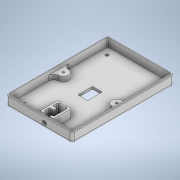
# Autodesk Inventor part: Controller_Back
Saved by Autodesk Inventor 2022.3 (Build 263350000, 350)
## iProperties
Created: 2023-06-20
Part Number: Controller_Back
Material: Generic
Document SubType Name: Modeling
Designer: natalie.jimenez
Density: 1 g/cm^3
Appearance: Default
Author: natalie.jimenez
Autodesk Inventor part; units mm, degrees
note: some values were not read from the file. Chosen so that the rebuilt part matches the saved one: direction of "Hole5"; direction of "Hole6".
ref_plane "YZ Plane" through (0, 0, 0) normal (1, 0, 0) x (0, 1, 0)
ref_plane "XZ Plane" through (0, 0, 0) normal (0, 1, 0) x (-1, 0, 0)
ref_plane "XY Plane" through (0, 0, 0) normal (0, 0, 1) x (1, 0, 0)
sketch "Sketch1" plane through (0, 0, 0) normal (0, 1, 0) x (-1, 0, 0)
  line L0 (40.64, -63.5) -> (-40.64, -63.5)
  line L1 (-40.64, -63.5) -> (-40.64, 63.5)
  line L2 (-40.64, 63.5) -> (40.64, 63.5)
  line L3 (40.64, 63.5) -> (40.64, -63.5)
  line L4 (40.64, -63.5) -> (-40.64, 63.5) construction
  line L5 (-40.64, -63.5) -> (40.64, 63.5) construction
  point P0 (0, 0)
  dimension "d0" = 127
  dimension "d1" = 81.28
  constraints: 12 end point, 2 midpoint, 2 parallel, 1 horizontal, 1 perpendicular
  measures "d0" distance between parallel lines of L0 L2
  measures "d1" distance between parallel lines of L1 L3
extrude "Extrusion1" add sketch "Sketch1" along normal blind 3.175
sketch "Sketch16" plane through (0, 0, 0) normal (0, -1, 0) x (1, 0, 0)
  line L0 (-42.672, -65.532) -> (42.672, -65.532)
  line L1 (42.672, -65.532) -> (42.672, 65.532)
  line L2 (42.672, 65.532) -> (-42.672, 65.532)
  line L3 (-42.672, 65.532) -> (-42.672, -65.532)
  line L4 (40.64, -63.5) -> (-40.64, -63.5) projected
  line L5 (-40.64, 63.5) -> (40.64, 63.5) projected
  line L6 (-40.64, -63.5) -> (-40.64, 63.5) projected
  line L7 (40.64, 63.5) -> (40.64, -63.5) projected
  point P0 (0, 0)
  dimension "d99" = 2.032
  dimension "d100" = 2.032
  dimension "d101" = 2.032
  dimension "d102" = 2.032
  constraints: 8 end point, 2 parallel, 1 horizontal, 1 perpendicular
  measures "d99" distance between parallel lines of L4 L0
  measures "d100" distance between parallel lines of L2 L5
  measures "d101" distance between parallel lines of L3 L6
  measures "d102" distance between parallel lines of L1 L7
extrude "Extrusion9" add sketch "Sketch16" against normal blind 12.7
fillet "Fillet1" radius 3.175 8 edges at (-42.672, 0, 0) (0, 0, 65.532) (42.672, 0, 0) (0, 0, -65.532) (-42.672, 6.35, -65.532) (42.672, 6.35, -65.532) (-42.672, 6.35, 65.532) (42.672, 6.35, 65.532)
fillet "Fillet3" radius 1.143 4 edges at (-40.64, 7.9375, -63.5) (40.64, 7.9375, -63.5) (-40.64, 7.9375, 63.5) (40.64, 7.9375, 63.5)
sketch "Sketch19" plane through (0, 12.7, 0) normal (0, 1, 0) x (1, 0, 0)
  arc A0 (-40.64, -62.357) -> (-39.497, -63.5) centre (-39.497, -62.357) ccw projected
  line L0 (39.497, -63.5) -> (-39.497, -63.5) projected
  line L1 (-40.64, -62.357) -> (-40.64, 62.357) projected
  arc A1 (-39.497, 63.5) -> (-40.64, 62.357) centre (-39.497, 62.357) ccw projected
  line L2 (-39.497, 63.5) -> (39.497, 63.5) projected
  arc A2 (40.64, 62.357) -> (39.497, 63.5) centre (39.497, 62.357) ccw projected
  line L3 (40.64, 62.357) -> (40.64, -62.357) projected
  arc A3 (39.497, -63.5) -> (40.64, -62.357) centre (39.497, -62.357) ccw projected
  line L4 (-41.656, 62.357) -> (-41.656, -62.357)
  arc A4 (-41.656, -62.357) -> (-39.497, -64.516) centre (-39.497, -62.357) ccw
  line L5 (-39.497, -64.516) -> (39.497, -64.516)
  arc A5 (39.497, -64.516) -> (41.656, -62.357) centre (39.497, -62.357) ccw
  line L6 (41.656, -62.357) -> (41.656, 62.357)
  arc A6 (41.656, 62.357) -> (39.497, 64.516) centre (39.497, 62.357) ccw
  line L7 (39.497, 64.516) -> (-39.497, 64.516)
  arc A7 (-39.497, 64.516) -> (-41.656, 62.357) centre (-39.497, 62.357) ccw
  point P0 (0, 0)
  dimension "d127" = 1.016
  constraints: 8 end point, 8 point on circle, 4 centre point, 7 other
  measures "d127" distance between parallel lines of L1 L4
extrude "Extrusion12" add sketch "Sketch19" along normal blind 1.27
sketch "Sketch20" plane through (0, 0, 0) normal (0, -1, 0) x (1, 0, 0)
  line L0 (-31.75, -53.721) -> (31.75, -53.721) construction
  line L1 (31.75, -53.721) -> (31.75, 53.721) construction
  line L2 (31.75, 53.721) -> (-31.75, 53.721) construction
  line L3 (-31.75, 53.721) -> (-31.75, -53.721) construction
  line L4 (-31.75, -53.721) -> (31.75, 53.721) construction
  line L5 (31.75, -53.721) -> (-31.75, 53.721) construction
  point P0 (0, 0)
  point P1 (31.75, -25.781)
  point P2 (31.75, 31.369)
  dimension "d130" = 57.15
  dimension "d131" = 63.5
  dimension "d132" = 107.442
  dimension "d207" = 27.94
  constraints: 12 end point, 2 coincident, 2 midpoint, 2 parallel, 2 point on line, 1 horizontal, 1 perpendicular
  measures "d130" distance of point (31.75, -25.781) point (31.75, 31.369)
  measures "d131" distance between parallel lines of L1 L3
  measures "d132" distance of point (-31.75, -53.721) L2.end
  measures "d207" vertical distance of point (31.75, -25.781) point (-31.75, -53.721)
sketch "Sketch21" plane through (0, 0, 0) normal (0, -1, 0) x (1, 0, 0)
  line L0 (-6.35, -9.525) -> (6.35, -9.525)
  line L1 (6.35, -9.525) -> (6.35, 9.525)
  line L2 (6.35, 9.525) -> (-6.35, 9.525)
  line L3 (-6.35, 9.525) -> (-6.35, -9.525)
  line L4 (-6.35, -9.525) -> (6.35, 9.525) construction
  line L5 (6.35, -9.525) -> (-6.35, 9.525) construction
  point P0 (0, 0)
  dimension "d133" = 12.7
  dimension "d134" = 19.05
  constraints: 12 end point, 2 midpoint, 2 parallel, 1 horizontal, 1 perpendicular
  measures "d133" distance between parallel lines of L1 L3
  measures "d134" distance between parallel lines of L0 L2
hole "Hole5" at (-31.75, 0, -53.721) at (31.75, 0, -25.781) at (31.75, 0, 31.369) at (-31.75, 0, 53.721) direction (0, 1, 0) diameter 3.81 depth 3.175 clearance for "Flat Head Machine Screw (82)" size "#6" standard "Ansi Unified Screw Threads"
extrude "Extrusion13" cut sketch "Sketch21" against normal up to surface (3.175 mm away)
fillet "Fillet4" radius 1.143 4 edges at (6.35, 1.5875, -9.525) (6.35, 1.5875, 9.525) (-6.35, 1.5875, 9.525) (-6.35, 1.5875, -9.525)
sketch "Sketch22" plane through (0, 0, 0) normal (0, -1, 0) x (1, 0, 0)
  line L0 (40.64, 62.357) -> (40.64, -62.357) projected
  line L1 (-40.64, -62.357) -> (-40.64, 62.357) projected
  line L2 (-59.7408, 0) -> (59.7408, 0) projected
  point P0 (0, 0)
  point P1 (34.29, 0)
  point P2 (-34.29, 0)
  point P3 (40.64, 0)
  point P4 (-40.64, 0)
  dimension "d147" = 6.35
  dimension "d148" = 6.35
  constraints: 2 midpoint, 2 point on line
  measures "d147" distance of point (40.64, 0) point (34.29, 0)
  measures "d148" distance of point (-34.29, 0) point (-40.64, 0)
hole "Hole6" at (-34.29, 0, 0) at (34.29, 0, 0) direction (0, 1, 0) diameter 2.6416 depth 3.175 thread size "6-32 UNC" class "2B" standard "ANSI Unified Screw Threads"
sketch "Sketch24" plane through (-39.497, 12.7, 65.532) normal (0, 0, 1) x (1, 0, 0)
  circle A0 centre (46.029, -6.6675) radius 2.8575
  line L0 (0, 0) -> (78.994, 0) projected
  line L1 (78.994, -9.525) -> (0, -9.525) projected
  line L2 (0, 0) -> (78.994, 0) projected
  line L3 (78.994, 0) -> (78.994, -9.525) projected
  point P0 (39.497, -12.7)
  point P1 (78.994, -4.7625)
  dimension "d157" = 5.715
  dimension "d159" = 33.02
  constraints: 1 centre point, 1 midpoint, 1 tangent
  measures "d157" diameter of A0
  measures "d159" distance of point (78.994, -4.763) A0.centre
extrude "Extrusion14" cut sketch "Sketch24" against normal up to surface (2.032 mm away)
sketch "Sketch25" plane through (0, 3.175, 0) normal (0, 1, 0) x (1, 0, 0)
  line L0 (3.6745, -63.5) -> (9.3895, -63.5) projected
  line L1 (-39.497, -62.357) -> (39.497, -62.357) projected
  line L2 (10.0245, -62.357) -> (15.7395, -62.357)
  line L3 (15.7395, -62.357) -> (15.7395, -39.497)
  line L4 (-2.0405, -39.497) -> (3.0395, -39.497)
  line L5 (15.7395, -62.357) -> (15.7395, -39.497)
  line L6 (-2.0405, -62.357) -> (-2.0405, -39.497)
  line L7 (15.7395, -39.497) -> (10.0245, -39.497)
  line L8 (10.0245, -39.497) -> (10.0245, -42.037)
  line L9 (10.0245, -42.037) -> (13.1995, -42.037)
  line L10 (0.4995, -42.037) -> (3.0395, -42.037)
  line L11 (3.0395, -42.037) -> (3.0395, -39.497)
  line L12 (15.7395, -62.357) -> (10.0245, -62.357)
  line L13 (10.0245, -62.357) -> (10.0245, -59.817)
  line L14 (10.0245, -59.817) -> (13.1995, -59.817)
  line L15 (3.0395, -62.357) -> (3.0395, -59.817)
  line L16 (3.0395, -59.817) -> (0.4995, -59.817)
  line L17 (0.4995, -52.832) -> (6.2145, -52.832)
  line L18 (6.2145, -52.832) -> (6.2145, -49.022)
  line L19 (6.2145, -49.022) -> (0.4995, -49.022)
  line L20 (39.497, -62.357) -> (39.497, 62.357) projected
  line L21 (15.7395, -39.497) -> (15.7395, -62.357)
  line L22 (10.0245, -62.357) -> (10.0245, -59.817)
  line L23 (0.4995, -49.022) -> (0.4995, -42.037)
  line L24 (0.4995, -52.832) -> (0.4995, -59.817)
  line L25 (10.0245, -40.767) -> (15.7395, -40.767) construction
  line L26 (10.0245, -61.087) -> (15.7395, -61.087) construction
  line L27 (13.1995, -42.037) -> (13.1995, -59.817)
  line L28 (-2.0405, -62.357) -> (3.0395, -62.357)
  line L29 (10.0245, -61.087) -> (3.0395, -61.087) construction
  line L30 (6.532, -63.5) -> (6.532, -61.087) construction
  point P0 (0, 0)
  point P1 (0.4995, -39.497)
  point P2 (12.882, -39.497)
  point P3 (-2.0405, -50.927)
  point P4 (0.4995, -56.3245)
  point P5 (3.0395, -40.767)
  dimension "d168" = 2.54
  dimension "d175" = 6.985
  dimension "d179" = 3.81
  dimension "d180" = 6.985
  dimension "d184" = 6.985
  dimension "d186" = 6.985
  dimension "d188" = 6.985
  dimension "d190" = 5.08
  dimension "d191" = 2.54
  dimension "d192" = 6.985
  dimension "d193" = 12.7
  dimension "d195" = 2.54
  dimension "d196" = 2.54
  dimension "d197" = 2.54
  constraints: 59 end point, 13 perpendicular, 10 midpoint, 8 parallel, 6 point on line, 4 horizontal, 2 collinear, 1 coincident, 2 other
  measures "d168" distance from line of L10 point (0.499, -39.497)
  measures "d175" distance between parallel lines of L8 L11
  measures "d179" distance between parallel lines of L17 L19
  measures "d180" distance of L26.start L29.end
  measures "d184" distance between parallel lines of L19 L10
  measures "d186" distance from line of L14 L17.end
  measures "d188" distance from line of L19 L8.end
  measures "d190" distance from line of point (3.039, -40.767) L6
  measures "d191" distance between parallel lines of L24 L6
  measures "d192" distance between parallel lines of L27 L18
  measures "d193" distance between parallel lines of L23 L27
  measures "d195" distance between parallel lines of L9 L7
  measures "d196" distance between parallel lines of L2 L14
  measures "d197" distance between parallel lines of L5 L27
extrude "Extrusion15" add sketch "Sketch25" along normal up to surface (10.795 mm away)
fillet "Fillet5" radius 1.27 20 edges at (15.7395, 8.5725, 39.497) (-2.0405, 8.5725, 39.497) (15.7395, 8.5725, 62.357) (-2.0405, 8.5725, 62.357) (6.2145, 8.5725, 49.022) (6.2145, 8.5725, 52.832) (0.4995, 8.5725, 42.037) (0.4995, 8.5725, 59.817) (13.1995, 8.5725, 59.817) (10.0245, 8.5725, 42.037) (10.0245, 8.5725, 39.497) (13.1995, 8.5725, 42.037) (10.0245, 8.5725, 59.817) (10.0245, 8.5725, 62.357) (3.0395, 8.5725, 42.037) (3.0395, 8.5725, 39.497) (3.0395, 8.5725, 59.817) (3.0395, 8.5725, 62.357) (0.4995, 8.5725, 52.832) (0.4995, 8.5725, 49.022)
sketch "Sketch26" plane through (0, 3.175, 0) normal (0, 1, 0) x (1, 0, 0)
  circle A0 centre (34.29, 0) radius 1.3208 projected
  arc A1 (34.29, 6.35) -> (34.29, -6.35) centre (34.29, 0) ccw
  circle A2 centre (-34.29, 0) radius 1.3208 projected
  arc A3 (-34.29, -6.35) -> (-34.29, 6.35) centre (-34.29, 0) ccw
  line L0 (40.64, -62.357) -> (40.64, 62.357) projected
  arc A4 (34.29, 6.35) -> (40.64, 12.7) centre (34.29, 12.7) ccw
  line L1 (-40.64, 62.357) -> (-40.64, -62.357) projected
  arc A5 (-40.64, 12.7) -> (-34.29, 6.35) centre (-34.29, 12.7) ccw
  line L2 (59.7408, 0) -> (-59.7408, 0) projected
  arc A6 (40.64, -12.7) -> (34.29, -6.35) centre (34.29, -12.7) ccw
  arc A7 (-34.29, -6.35) -> (-40.64, -12.7) centre (-34.29, -12.7) ccw
  point P0 (0, 0)
  point P1 (-40.64, -12.7)
  point P2 (40.64, -12.7)
  dimension "d201" = 12.7
  dimension "d202" = 12.7
  dimension "d203" = 6.35
  dimension "d204" = 6.35
  constraints: 12 point on circle, 6 centre point, 6 symmetric about line, 4 tangent, 2 coincident, 2 point on line, 2 other
  measures "d201" diameter of A3
  measures "d202" diameter of A1
  measures "d203" radius of A4
  measures "d204" radius of A5
extrude "Extrusion16" add sketch "Sketch26" along normal blind 6.35 contours L2 L0 A6 A1 A0 | A0 L2 A1 A4 L0 | L2 A3 A7 L1 A2 | A2 L2 L1 A5 A3
sketch "Sketch2" plane through (0, 3.175, 0) normal (0, 1, 0) x (1, 0, 0)
  line L0 (11.7475, 17.4625) -> (-11.7475, 17.4625)
  line L1 (-11.7475, 17.4625) -> (-11.7475, -17.4625)
  line L2 (-11.7475, -17.4625) -> (11.7475, -17.4625)
  line L3 (11.7475, -17.4625) -> (11.7475, 17.4625)
  line L4 (11.7475, 17.4625) -> (-11.7475, -17.4625) construction
  line L5 (-11.7475, 17.4625) -> (11.7475, -17.4625) construction
  point P0 (0, 0)
  dimension "d4" = 23.495
  dimension "d5" = 34.925
  constraints: 12 end point, 2 midpoint, 2 parallel, 1 horizontal, 1 perpendicular
  measures "d4" distance between parallel lines of L3 L1
  measures "d5" distance between parallel lines of L0 L2
sketch "Sketch4" plane through (0, 0, 0) normal (0, 0, 1) x (1, 0, 0)
  line L0 (11.7475, 1.143) -> (17.3304, 3.175)
  line L1 (40.64, 3.175) -> (-40.64, 3.175) projected
  line L2 (11.7475, 3.175) -> (11.7475, 1.143) projected
  line L3 (11.7475, 1.143) -> (11.7475, 3.175)
  line L4 (11.7475, 3.175) -> (17.3304, 3.175)
  point P0 (0, 0)
  dimension "d8" = 70
  constraints: 6 end point, 1 collinear, 1 perpendicular, 1 point on line
  measures "d8" angle of L2 L0
sketch "Sketch5" plane through (0, 0, 0) normal (0, 0, 1) x (1, 0, 0)
  line L0 (-11.7475, 1.143) -> (11.7475, 1.143) projected
  line L1 (40.64, 3.175) -> (-40.64, 3.175) projected
  line L2 (-11.7475, 1.143) -> (-16.8275, 1.143)
  line L3 (-16.8275, 1.143) -> (-16.8275, 3.175)
  line L4 (-16.8275, 3.175) -> (-11.7475, 3.175)
  line L5 (-11.7475, 3.175) -> (-11.7475, 1.143)
  point P0 (0, 0)
  point P1 (-11.7475, 2.159)
  point P2 (-16.8275, 2.159)
  dimension "d11" = 5.08
  constraints: 8 end point, 2 midpoint, 2 parallel, 1 horizontal, 1 perpendicular, 1 point on line
  measures "d11" distance of point (-11.748, 2.159) point (-16.828, 2.159)
sketch "Sketch6" plane through (0, 1.143, 0) normal (0, 1, 0) x (1, 0, 0)
  line L0 (-11.7475, -17.4625) -> (-11.7475, -7.62) projected
  line L1 (11.7475, -17.4625) -> (-11.7475, -17.4625) projected
  line L2 (11.7475, -7.62) -> (11.7475, -17.4625) projected
  line L3 (11.7475, 7.62) -> (11.7475, -7.62) projected
  line L4 (11.7475, 17.4625) -> (11.7475, 7.62) projected
  line L5 (-11.7475, 17.4625) -> (11.7475, 17.4625) projected
  line L6 (-11.7475, 7.62) -> (-11.7475, 17.4625) projected
  line L7 (-11.7475, 7.62) -> (-16.8275, 7.62) projected
  line L8 (-16.8275, 7.62) -> (-16.8275, -7.62) projected
  line L9 (-16.8275, -7.62) -> (-11.7475, -7.62) projected
  line L10 (-10.6045, 16.0655) -> (6.9215, 16.0655)
  line L11 (6.9215, 16.0655) -> (6.9215, -16.0655)
  line L12 (6.9215, -16.0655) -> (-10.6045, -16.0655)
  line L13 (-10.6045, -16.0655) -> (-10.6045, 16.0655)
  line L14 (11.7475, 7.62) -> (11.7475, -7.62) projected
  line L15 (11.7475, 0) -> (-16.8275, 0) construction
  line L16 (-16.8275, -7.62) -> (-16.8275, 7.62) projected
  line L17 (6.9215, 0) -> (-10.6045, 0) construction
  point P0 (0, 0)
  dimension "d14" = 17.526
  dimension "d15" = 32.131
  dimension "d16" = 4.826
  constraints: 12 end point, 4 midpoint, 2 parallel, 1 collinear, 1 horizontal, 1 perpendicular
  measures "d14" distance between parallel lines of L11 L13
  measures "d15" distance between parallel lines of L12 L10
  measures "d16" distance between parallel lines of L3 L11
sketch "Sketch7" plane through (0, 3.175, 0) normal (0, 1, 0) x (1, 0, 0)
  line L0 (-14.2875, 12.7) -> (13.6525, 12.7) construction
  line L1 (13.6525, 12.7) -> (13.6525, -12.7) construction
  line L2 (13.6525, -12.7) -> (-14.2875, -12.7) construction
  line L3 (-14.2875, -12.7) -> (-14.2875, 12.7) construction
  line L4 (-10.6045, -16.0655) -> (-10.6045, 16.0655) projected
  line L5 (-14.2875, 0) -> (13.6525, 0) construction
  line L6 (-10.6045, 0) -> (6.9215, 0) construction
  line L7 (6.9215, 16.0655) -> (6.9215, -16.0655) projected
  line L8 (-11.7475, 7.62) -> (-11.7475, 17.4625) projected
  point P0 (0, 0)
  dimension "d19" = 25.4
  dimension "d20" = 27.94
  dimension "d21" = 2.54
  constraints: 12 end point, 4 midpoint, 3 parallel, 1 collinear, 1 horizontal
  measures "d19" distance of L2.end L0.start
  measures "d20" distance between parallel lines of L1 L3
  measures "d21" distance between parallel lines of L3 L8
sketch "Sketch8" plane through (0, 3.175, 0) normal (0, 1, 0) x (1, 0, 0)
  line L0 (-37.1182, -59.7067) -> (-16.7982, -59.7067)
  line L1 (-16.7982, -59.7067) -> (-16.7982, -21.7067)
  line L2 (-16.7982, -21.7067) -> (-37.1182, -21.7067)
  line L3 (-37.1182, -21.7067) -> (-37.1182, -59.7067)
  point P0 (0, 0)
  dimension "d29" = 20.32
  dimension "d30" = 38
  constraints: 8 end point, 2 parallel, 1 horizontal, 1 perpendicular
  measures "d29" distance between parallel lines of L3 L1
  measures "d30" distance between parallel lines of L2 L0
sketch "Sketch11" plane through (0, 3.175, 0) normal (0, 1, 0) x (1, 0, 0)
  line L0 (-34.5782, -61.0275) -> (-19.3382, -61.0275) construction
  line L1 (-16.7982, -59.7067) -> (-37.1182, -59.7067) projected
  line L2 (-19.3382, -61.0275) -> (-19.3382, -20.3875) construction
  line L3 (-19.3382, -20.3875) -> (-34.5782, -20.3875) construction
  line L4 (-34.5782, -20.3875) -> (-34.5782, -61.0275) construction
  line L5 (-37.1182, -21.7067) -> (-16.7982, -21.7067) projected
  line L6 (-37.1182, -59.7067) -> (-37.1182, -21.7067) projected
  line L7 (-16.7982, -21.7067) -> (-16.7982, -59.7067) projected
  line L8 (-16.7982, -59.7067) -> (-37.1182, -59.7067) projected
  line L9 (-16.7982, -21.7067) -> (-16.7982, -59.7067) projected
  line L10 (-37.1182, -21.7067) -> (-16.7982, -21.7067) projected
  line L11 (-37.1182, -59.7067) -> (-37.1182, -21.7067) projected
  line L12 (-16.7982, -59.7067) -> (-37.1182, -59.7067) projected
  line L13 (-34.5782, -40.7075) -> (-37.1182, -40.7067)
  line L14 (-37.1182, -59.7067) -> (-37.1182, -21.7067) projected
  line L15 (-19.3382, -40.7075) -> (-16.7982, -40.7067)
  line L16 (-16.7982, -21.7067) -> (-16.7982, -59.7067) projected
  point P0 (0, 0)
  dimension "d38" = 15.24
  dimension "d39" = 40.64
  dimension "d40" = 1.3208
  constraints: 12 end point, 5 parallel, 4 midpoint, 3 perpendicular, 1 equal length
  measures "d38" distance from line of L0.end L4
  measures "d39" distance between parallel lines of L3 L0
  measures "d40" distance between parallel lines of L1 L0
sketch "Sketch12" plane through (0, 3.175, 0) normal (0, 1, 0) x (1, 0, 0)
  line L0 (-7.747, 38.227) -> (37.719, 38.227) construction
  line L1 (37.719, 38.227) -> (37.719, 59.309) construction
  line L2 (37.719, 59.309) -> (-7.747, 59.309) construction
  line L3 (-7.747, 59.309) -> (-7.747, 38.227) construction
  line L4 (-0.508, 57.15) -> (30.48, 57.15) construction
  line L5 (30.48, 57.15) -> (30.48, 40.386) construction
  line L6 (30.48, 40.386) -> (-0.508, 40.386) construction
  line L7 (-0.508, 40.386) -> (-0.508, 57.15) construction
  line L8 (-40.64, -63.5) -> (40.64, -63.5) projected
  line L9 (40.64, -63.5) -> (40.64, 63.5) projected
  line L10 (-0.508, 48.768) -> (-7.747, 48.768) construction
  line L11 (30.48, 48.768) -> (37.719, 48.768) construction
  line L12 (40.64, 63.5) -> (-40.64, 63.5) projected
  point P0 (0, 0)
  dimension "d49" = 21.082
  dimension "d63" = 16.764
  dimension "d64" = 30.988
  dimension "d114" = 6.35
  dimension "d115" = 10.16
  constraints: 20 end point, 4 midpoint, 4 parallel, 3 perpendicular, 2 horizontal, 1 collinear
  measures "d49" distance between parallel lines of L2 L0
  measures "d63" distance between parallel lines of L4 L6
  measures "d64" distance between parallel lines of L5 L7
  measures "d114" distance between parallel lines of L12 L4
  measures "d115" distance between parallel lines of L9 L5
sketch "Sketch13" plane through (0, 3.175, 0) normal (0, 1, 0) x (1, 0, 0)
  circle A0 centre (18.161, -40.64) radius 9.525
  line L0 (40.64, -63.5) -> (40.64, 63.5) projected
  line L1 (40.64, 63.5) -> (-40.64, 63.5) projected
  line L2 (26.924, -44.373) -> (26.924, -36.907)
  line L3 (8.636, -40.64) -> (26.924, -40.64) construction
  line L4 (-40.64, -63.5) -> (40.64, -63.5) projected
  point P0 (0, 0)
  point P1 (17.78, -40.64)
  dimension "d65" = 19.05
  dimension "d98" = 18.288
  dimension "d116" = 22.86
  dimension "d117" = 22.86
  constraints: 4 end point, 3 point on circle, 2 midpoint, 1 centre point, 1 vertical
  measures "d65" diameter of A0
  measures "d98" distance of L3.start L3.end
  measures "d116" distance from line of L4 point (17.78, -40.64)
  measures "d117" distance from line of L0 point (17.78, -40.64)
sketch "Sketch14" plane through (0, 3.175, 0) normal (0, 1, 0) x (1, 0, 0)
  line L0 (-35.56, 58.42) -> (-21.463, 58.42) construction
  line L1 (-21.463, 58.42) -> (-21.463, 13.97) construction
  line L2 (-21.463, 13.97) -> (-35.56, 13.97) construction
  line L3 (-35.56, 13.97) -> (-35.56, 58.42) construction
  line L4 (-35.56, 13.97) -> (-21.463, 13.97)
  line L5 (-21.463, 13.97) -> (-21.463, 17.145)
  line L6 (-21.463, 17.145) -> (-35.56, 17.145)
  line L7 (-35.56, 17.145) -> (-35.56, 13.97)
  line L8 (-35.56, 58.42) -> (-21.463, 58.42)
  line L9 (-21.463, 58.42) -> (-21.463, 55.245)
  line L10 (-21.463, 55.245) -> (-35.56, 55.245)
  line L11 (-35.56, 55.245) -> (-35.56, 58.42)
  line L12 (-40.64, 63.5) -> (-40.64, -63.5) projected
  line L13 (40.64, 63.5) -> (-40.64, 63.5) projected
  point P0 (0, 0)
  point P1 (-35.56, 15.5575)
  point P2 (-28.5115, 58.42)
  dimension "d72" = 44.45
  dimension "d73" = 14.097
  dimension "d74" = 3.175
  dimension "d75" = 3.175
  dimension "d76" = 5.08
  dimension "d77" = 5.08
  constraints: 24 end point, 6 parallel, 3 horizontal, 3 perpendicular, 2 midpoint, 2 point on line
  measures "d72" distance between parallel lines of L2 L0
  measures "d73" distance between parallel lines of L3 L1
  measures "d74" distance between parallel lines of L6 L2
  measures "d75" distance between parallel lines of L0 L10
  measures "d76" distance from line of L12 point (-35.56, 15.557)
  measures "d77" distance from line of L13 point (-28.512, 58.42)
sketch "Sketch15" plane through (0, 3.175, 0) normal (0, 1, 0) x (1, 0, 0)
  line L0 (-35.56, 13.97) -> (-35.56, 17.145) projected
  line L1 (-35.56, 58.42) -> (-21.463, 58.42) construction
  line L2 (-35.56, 13.97) -> (-21.463, 13.97)
  line L3 (-21.463, 13.97) -> (-21.463, 58.42) construction
  line L4 (-21.463, 58.42) -> (-35.56, 58.42)
  line L5 (-35.56, 58.42) -> (-35.56, 13.97) construction
  line L6 (-38.1, 33.02) -> (-18.923, 33.02) construction
  line L7 (-18.923, 39.37) -> (-38.1, 39.37) construction
  line L8 (-21.463, 55.245) -> (-35.56, 55.245) projected
  line L9 (-35.56, 17.145) -> (-21.463, 17.145) projected
  line L10 (-28.5115, 17.145) -> (-28.5115, 33.02) construction
  line L11 (-28.5115, 39.37) -> (-28.5115, 55.245) construction
  point P0 (0, 0)
  point P1 (-38.1, 39.37)
  dimension "d85" = 6.35
  dimension "d86" = 6.35
  dimension "d89" = 19.05
  dimension "d90" = 19.05
  dimension "d118" = 2.54
  dimension "d119" = 2.54
  dimension "d120" = 2.54
  constraints: 16 end point, 4 midpoint, 3 parallel, 2 horizontal, 1 coincident, 1 equal length, 1 perpendicular
  measures "d85" distance of point (-38.1, 39.37) L6.start
  measures "d86" distance of L7.start L6.end
  measures "d89" distance between parallel lines of L1 L7
  measures "d90" distance between parallel lines of L2 L6
  measures "d118" distance from line of L6.start L5
  measures "d119" distance from line of point (-38.1, 39.37) L5
  measures "d120" distance from line of L3 L6.end
sketch "Sketch17" plane through (-42.672, 0, 65.532) normal (0, 0, 1) x (1, 0, 0)
  line L0 (25.8738, 3.175) -> (5.5538, 3.175) construction
  line L1 (21.209, 3.175) -> (7.112, 3.175) projected
  line L2 (83.312, 12.7) -> (2.032, 12.7) projected
  line L3 (12.8022, 3.175) -> (10.2528, 3.175)
  line L4 (10.2528, 3.175) -> (10.2528, 8.509)
  line L5 (12.8022, 3.175) -> (21.1748, 3.175)
  line L6 (21.1748, 3.175) -> (21.1748, 8.509)
  line L7 (21.209, 3.175) -> (7.112, 3.175) projected
  line L8 (10.2528, 8.509) -> (21.1748, 8.509)
  line L9 (5.5538, 3.175) -> (10.2528, 8.509) construction
  line L10 (5.5538, 3.175) -> (25.8738, 3.175) projected
  line L11 (21.1748, 8.509) -> (25.8738, 3.175) construction
  line L12 (25.8738, 1.524) -> (5.5538, 1.524) projected
  line L13 (3.175, 12.7) -> (82.169, 12.7) projected
  line L14 (21.1748, 8.509) -> (21.1748, 3.175)
  line L15 (82.169, 12.7) -> (82.169, 3.175) projected
  line L16 (3.175, 3.175) -> (3.175, 12.7) projected
  line L17 (82.169, 3.175) -> (3.175, 3.175) projected
  point P0 (42.672, 0)
  point P1 (11.5275, 3.175)
  point P2 (10.2528, 5.842)
  point P3 (10.2528, 3.175)
  dimension "d109" = 10.922
  dimension "d110" = 5.334
  constraints: 16 end point, 5 perpendicular, 2 equal length, 2 horizontal, 2 midpoint, 1 point on line
  measures "d109" distance of L4.end L6.end
  measures "d110" distance between parallel lines of L8 L0
sketch "Sketch18" plane through (0, 12.7, 0) normal (0, 1, 0) x (1, 0, 0)
  line L0 (-39.497, -65.532) -> (39.497, -65.532) projected
  arc A0 (-42.672, -62.357) -> (-39.497, -65.532) centre (-39.497, -62.357) ccw projected
  line L1 (-42.672, 62.357) -> (-42.672, -62.357) projected
  arc A1 (-39.497, 65.532) -> (-42.672, 62.357) centre (-39.497, 62.357) ccw projected
  line L2 (39.497, 65.532) -> (-39.497, 65.532) projected
  arc A2 (42.672, 62.357) -> (39.497, 65.532) centre (39.497, 62.357) ccw projected
  line L3 (42.672, -62.357) -> (42.672, 62.357) projected
  arc A3 (39.497, -65.532) -> (42.672, -62.357) centre (39.497, -62.357) ccw projected
  arc A4 (-41.656, -62.357) -> (-39.497, -64.516) centre (-39.497, -62.357) ccw
  line L4 (-39.497, -64.516) -> (39.497, -64.516)
  arc A5 (39.497, -64.516) -> (41.656, -62.357) centre (39.497, -62.357) ccw
  line L5 (41.656, -62.357) -> (41.656, 62.357)
  arc A6 (41.656, 62.357) -> (39.497, 64.516) centre (39.497, 62.357) ccw
  line L6 (39.497, 64.516) -> (-39.497, 64.516)
  arc A7 (-39.497, 64.516) -> (-41.656, 62.357) centre (-39.497, 62.357) ccw
  line L7 (-41.656, 62.357) -> (-41.656, -62.357)
  point P0 (0, 0)
  dimension "d123" = 1.016
  constraints: 8 end point, 8 point on circle, 4 centre point, 7 other
  measures "d123" distance between parallel lines of L1 L7
equation "\"d148\" = d147"
body "Solid1"
